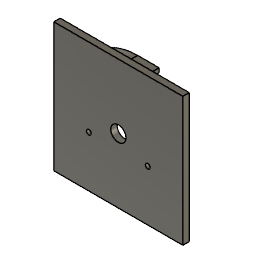
stepper motor base v1 (Autodesk Fusion 360 design; units mm, degrees)
part number: 2026-04-22-00-17-38-220
Autodesk Fusion 360 part; units mm, degrees
sketch "Sketch1" plane through (0, 0, 0) normal (0, 1, 0) x (1, 0, 0)
  line L0 (38.1, 38.1) -> (-38.1, 38.1)
  line L1 (-38.1, 38.1) -> (-38.1, -38.1)
  line L2 (-38.1, -38.1) -> (38.1, -38.1)
  line L3 (38.1, -38.1) -> (38.1, 38.1)
  line L4 (38.1, 38.1) -> (-38.1, -38.1) construction
  line L5 (-38.1, 38.1) -> (38.1, -38.1) construction
  dimension "d1" = 76.2
  dimension "d2" = 76.2
  constraint horizontal L0
  constraint perpendicular L0 L1
  constraint parallel L0 L2
  constraint parallel L1 L3
  constraint coincident L4 origin
  constraint coincident L5 origin
  measures "d1" distance of L1.end L2.end
  measures "d2" distance of L0.end L1.end
extrude "Extrude1" add sketch "Sketch1" along normal blind 3.81
sketch "Sketch2" plane through (0, 3.81, 0) normal (0, 1, 0) x (-1, 0, 0)
  line L0 (-38.1, 38.1) -> (-38.1, -38.1)
  line L1 (-38.1, -38.1) -> (38.1, -38.1)
  line L2 (38.1, -38.1) -> (38.1, 38.1)
  line L3 (38.1, 38.1) -> (-38.1, 38.1)
  circle A0 centre (-17.399, -8) radius 1.4
  circle A1 centre (17.399, -8) radius 1.4
  line L4 (0, 1.75) -> (0, 22.5)
  circle A2 centre (0, 0) radius 4.5
  line L5 (-50.0726, -8) -> (46.4474, -8) construction
  dimension "d5" = 34.798
  dimension "d6" = 2.8
  dimension "d7" = 2.8
  dimension "d8" = 9
  dimension "d9" = 8
  constraint symmetric A0.centre A1.centre L4
  constraint coincident L4 A2.centre
  constraint horizontal L5
  constraint coincident A2.centre origin
  constraint coincident A0.centre L5
  measures "d5" distance of A0.centre A1.centre
  measures "d6" diameter of A0
  measures "d7" diameter of A1
  measures "d8" diameter of A2
  measures "d9" distance of A2.centre L5
extrude "Extrude2" cut sketch "Sketch2" against normal through all contours A0 | A1 | A2
sketch "Sketch3" plane through (0, 3.81, 0) normal (0, 1, 0) x (-1, 0, 0)
  circle A0 centre (0, 0) radius 4.5
  circle A1 centre (-17.399, -8) radius 1.4
  circle A2 centre (17.399, -8) radius 1.4
  line L0 (-38.1, 38.1) -> (-38.1, -38.1)
  line L1 (-38.1, -38.1) -> (38.1, -38.1)
  line L2 (38.1, -38.1) -> (38.1, 38.1)
  line L3 (38.1, 38.1) -> (-38.1, 38.1)
  line L4 (0, 44.3572) -> (0, -39.4628) construction
  line L5 (0, 1.75) -> (0, 22.5)
  arc A3 (0, -31.75) -> (0, 31.75) centre (0, 0) ccw
  arc A4 (0, -34.29) -> (0, 34.29) centre (0, 0) ccw
  line L6 (0, 34.29) -> (-12.7, 34.29)
  line L7 (-12.7, 34.29) -> (-12.7, 31.75)
  line L8 (-12.7, 31.75) -> (0, 31.75)
  line L9 (0, -31.75) -> (-12.7, -31.75)
  line L10 (-12.7, -31.75) -> (-12.7, -34.29)
  line L11 (-12.7, -34.29) -> (0, -34.29)
  dimension "d11" = 63.5
  dimension "d12" = 68.58
  dimension "d13" = 12.7
  dimension "d14" = 12.7
  constraint concentric A0 A3
  constraint concentric A3 A4
  constraint parallel L0 L4
  constraint collinear L4 L5
  constraint coincident L4 A3.end
  constraint coincident L4 A3.start
  constraint coincident L4 A4.end
  constraint coincident L4 A4.start
  constraint tangent A4 L6
  constraint perpendicular L6 L7
  constraint tangent A3 L8
  constraint tangent A3 L9
  constraint perpendicular L9 L10
  constraint tangent A4 L11
  measures "d11" diameter of A3
  measures "d12" diameter of A4
  measures "d13" distance of L4 L7
  measures "d14" distance of L4 L10
extrude "Extrude3" add sketch "Sketch3" along normal blind 7.62 contours A3 A4 L6 L7 L8 L9 L10 L11
